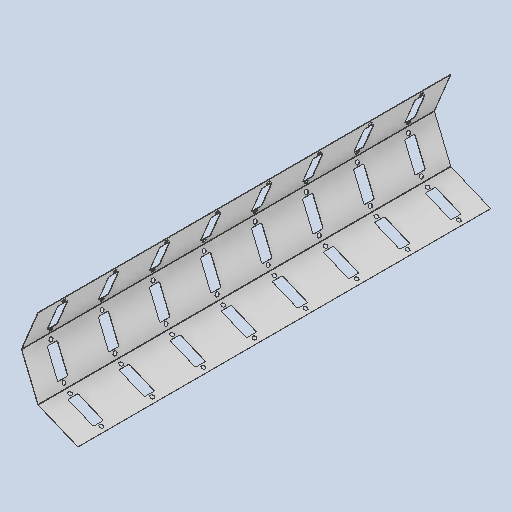
# Autodesk Inventor part: ДМФ 01 13 Барабан Лист лев брт
Saved by Autodesk Inventor 2024.2 (Build 282272000, 272)
## iProperties
Created: 2024-04-28
Part Number: ДМФ 01 13 Барабан Лист лев брт
Material: Generic
Document SubType Name: Sheet Metal
Designer: pokla
Density: 1 g/cm^3
Appearance: Default
Sheet Metal Rule: Default
Flat Pattern Width: 63.3571 cm
Flat Pattern Length: 202 cm
Flat Pattern Area: 12798.1 cm^2
Sheet Metal Width: 633,571 mm
Sheet Metal Length: 2020,000 mm
Sheet Metal Area: 1279813,721 mm^2
Stock Number: Барабан_Лист_Левый_Борт
Author: pokla
Autodesk Inventor part; units mm, degrees
ref_plane "YZ Plane" through (0, 0, 0) normal (1, 0, 0) x (0, 1, 0)
ref_plane "XZ Plane" through (0, 0, 0) normal (0, 1, 0) x (-1, 0, 0)
ref_plane "XY Plane" through (0, 0, 0) normal (0, 0, 1) x (1, 0, 0)
sketch "Sketch2" plane through (0, 0, 0) normal (0, 0, 1) x (1, 0, 0)
  line L0 (0, 277.6336) -> (196.3166, 196.3166) construction
  line L1 (196.3166, 196.3166) -> (277.6336, 0) construction
  line L2 (277.6336, 0) -> (196.3166, -196.3166) construction
  line L3 (196.3166, -196.3166) -> (0, -277.6336) construction
  line L4 (0, -277.6336) -> (-196.3166, -196.3166) construction
  line L5 (-196.3166, -196.3166) -> (-277.6336, 0) construction
  line L6 (-277.6336, 0) -> (-196.3166, 196.3166) construction
  line L7 (-196.3166, 196.3166) -> (0, 277.6336) construction
  line L8 (-276.9995, -1.5307) -> (-196.9507, -194.7859)
  line L9 (-194.7859, -196.9507) -> (-0.8315, -277.2892)
  arc A0 (-276.9995, 1.5307) -> (-276.9995, -1.5307) centre (-273.304, 0) ccw
  arc A1 (-196.9507, -194.7859) -> (-194.7859, -196.9507) centre (-193.2551, -193.2551) ccw
  line L10 (-276.9995, 1.5307) -> (-196.661, 195.4851)
  point P0 (0, 0)
  point P1 (0, 0)
  dimension "d58" = 4
  dimension "d59" = 4
  dimension "d70" = 0.9
  dimension "d72" = 0.9
  dimension "d74" = 513
  measures "d58" radius of A0
  measures "d59" radius of A1
  measures "d70" distance of L3.end L9.end
  measures "d72" distance of L6.end L10.end
  measures "d74" distance between parallel lines of L1 L8
contour flange "Contour Flange3" sketch "Sketch2" thickness 2 bend radius 2 width 2020 along (0, 0, -1) mid plane no both sides no wall seen from (-97.8087, -237.1199, 0) lies toward (0.3826834, 0.9238795, 0) curves L9 A1 L8 A0 L10
bend "Bend6"
corner "Corner6"
sketch "Sketch11" plane through (-275.1518, -0.7654, 0) normal (0.9238795, 0.3826834, 0) x (0, 0, -1)
  line L0 (0, 0) -> (2020, 0) projected
  line L1 (0, -209.1778) -> (0, 0) projected
  line L2 (0, -209.1778) -> (2020, -209.1778) projected
  line L3 (2020, -209.1778) -> (2020, 0) projected
  line L4 (860, -37.0889) -> (910, -37.0889)
  line L5 (910, -37.0889) -> (910, -172.0889)
  line L6 (910, -172.0889) -> (860, -172.0889)
  line L7 (860, -172.0889) -> (860, -37.0889)
  line L8 (860, -104.5889) -> (910, -104.5889) construction
  line L9 (885, -22.0889) -> (885, -187.0889) construction
  line L10 (880.1503, -30.4889) -> (875.3005, -22.0889)
  line L11 (875.3005, -22.0889) -> (880.1503, -13.6889)
  line L12 (880.1503, -13.6889) -> (889.8497, -13.6889)
  line L13 (889.8497, -13.6889) -> (894.6995, -22.0889)
  line L14 (894.6995, -22.0889) -> (889.8497, -30.4889)
  line L15 (889.8497, -30.4889) -> (880.1503, -30.4889)
  line L16 (889.8497, -178.6889) -> (894.6995, -187.0889)
  line L17 (894.6995, -187.0889) -> (889.8497, -195.4889)
  line L18 (889.8497, -195.4889) -> (880.1503, -195.4889)
  line L19 (880.1503, -195.4889) -> (875.3005, -187.0889)
  line L20 (875.3005, -187.0889) -> (880.1503, -178.6889)
  line L21 (880.1503, -178.6889) -> (889.8497, -178.6889)
  point P0 (0, -104.5889)
  point P1 (2020, -104.5889)
  point P2 (885, -37.0889)
  point P3 (885, -172.0889)
  point P4 (1010, 0)
  point P5 (885, -30.4889)
  point P6 (885, -178.6889)
  point P7 (885, -104.5889)
  dimension "d141" = 50
  dimension "d142" = 135
  dimension "d145" = 125
  dimension "d159" = 16.8
  dimension "d160" = 16.8
  dimension "d161" = 165
  constraints: 36 end point, 10 midpoint, 2 coincident, 2 horizontal, 2 parallel, 2 point on line, 2 vertical alignment, 1 horizontal alignment, 1 perpendicular, 1 vertical, 26 other
  measures "d141" distance of L4.start L4.end
  measures "d142" distance of L4.end L5.end
  measures "d145" horizontal distance of L9.start point (1010, 0)
  measures "d159" distance between parallel lines of L15 L12
  measures "d160" distance between parallel lines of L18 L21
  measures "d161" distance of L9.start L9.end
extrude "Extrusion4" cut sketch "Sketch11" against normal blind 10 contours L4 L5 L6 L7 | L10 L11 L12 L13 L14 L15 | L16 L17 L18 L19 L20 L21
fillet "Fillet1" radius 5 4 edges at (-261.8824, -35.4137, -910) (-261.8824, -35.4137, -860) (-210.2201, -160.1375, -860) (-210.2201, -160.1375, -910)
pattern_circular "Circular Pattern2" count 3 over 90 about axis through (0, 0, -10) along (0, 0, 1) of "Extrusion4", "Fillet1" both ways yes
pattern_linear "Rectangular Pattern2" count 8 spacing 250 along (0, 0, -1) of "Extrusion4", "Fillet1", "Circular Pattern2" first direction both ways yes
fillet "Corner Round1" radius 2 1 edges at (-195.7371, 195.1024, -2020)
sketch "Sketch11:Copy" plane through (0, 0, -2) normal (0, 0, -1) x (1, 0, 0)
  line L0 (0, 0) -> (2020, 0) projected
  line L1 (0, -209.1778) -> (0, 0) projected
  line L2 (0, -209.1778) -> (2020, -209.1778) projected
  line L3 (2020, -209.1778) -> (2020, 0) projected
  line L4 (860, -37.0889) -> (910, -37.0889) projected
  line L5 (910, -37.0889) -> (910, -172.0889) projected
  line L6 (910, -172.0889) -> (860, -172.0889) projected
  line L7 (860, -172.0889) -> (860, -37.0889) projected
  line L8 (860, -104.5889) -> (910, -104.5889) construction
  line L9 (885, -22.0889) -> (885, -187.0889) construction
  line L10 (880.1503, -30.4889) -> (875.3005, -22.0889) projected
  line L11 (875.3005, -22.0889) -> (880.1503, -13.6889) projected
  line L12 (880.1503, -13.6889) -> (889.8497, -13.6889) projected
  line L13 (889.8497, -13.6889) -> (894.6995, -22.0889) projected
  line L14 (894.6995, -22.0889) -> (889.8497, -30.4889) projected
  line L15 (889.8497, -30.4889) -> (880.1503, -30.4889) projected
  line L16 (889.8497, -178.6889) -> (894.6995, -187.0889) projected
  line L17 (894.6995, -187.0889) -> (889.8497, -195.4889) projected
  line L18 (889.8497, -195.4889) -> (880.1503, -195.4889) projected
  line L19 (880.1503, -195.4889) -> (875.3005, -187.0889) projected
  line L20 (875.3005, -187.0889) -> (880.1503, -178.6889) projected
  line L21 (880.1503, -178.6889) -> (889.8497, -178.6889) projected
  point P0 (0, -104.5889)
  point P1 (2020, -104.5889)
  point P2 (885, -37.0889)
  point P3 (885, -172.0889)
  point P4 (1010, 0)
  point P5 (885, -30.4889)
  point P6 (885, -178.6889)
  point P7 (885, -104.5889)
  constraints: 2 other
equation "\"d58\" = BendRadius + Thickness"
equation "\"d59\" = BendRadius + Thickness"
equation "\"d74\" = Барабан_габарит_по_кассетам"
equation "\"d75\" = Thickness"
equation "\"d76\" = BendReliefWidth"
equation "\"d77\" = BendReliefDepth"
equation "\"d78\" = MinimumRemnant"
equation "\"d79\" = TransitionRadius"
equation "\"d80\" = Барабан_длина_листа"
equation "\"d81\" = BendRadius"
equation "\"d83\" = CornerReliefSize"
equation "\"d84\" = GapSize"
equation "\"d85\" = JacobiRadiusSize"
equation "\"BendRadius\" = Thickness"
equation "\"BendReliefWidth\" = Thickness"
equation "\"BendReliefDepth\" = 0.5 * Thickness"
equation "\"CornerReliefSize\" = 4 * Thickness"
equation "\"MinimumRemnant\" = 2 * Thickness"
equation "\"TransitionRadius\" = BendRadius"
equation "\"JacobiRadiusSize\" = BendRadius"
equation "\"GapSize\" = Thickness"
equation "\"Барабан_Середина_листа\" = 206.27835"
equation "\"Thickness\" = 2"
equation "\"Барабан_габарит_по_кассетам\" = 513"
equation "\"Барабан_длина_листа\" = 2020"
body "Solid3"
